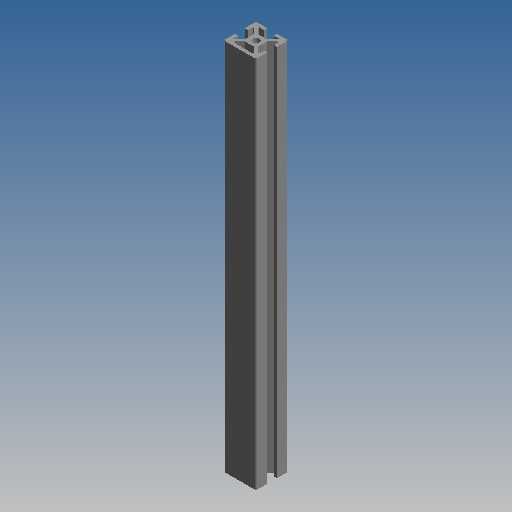
# Autodesk Inventor part: NFSF5-2020-231
Saved by Autodesk Inventor 2020 (Build 240168000, 168)
## iProperties
Part Number: NFSF5-2020-231
Material: 一般
Catalog Web Link: www.cadenas.de
Description: NFS5-2020, NFSB5-2020, HFS5-2020, HFSB5-2020, CAF5-2020, HFSY5-2020, NFSF5-2020, HFSF5-2020, HFSFB5-2020, NFST5-2020, HFST5-2020, HFSTB5-2020, HFSH5-2020, HFSC5-2020-HFS5 Series Aluminum Extrusions 20 Square -1 Slot-
Vendor: MISUMI
Document SubType Name: Modeling
Designer: partserver
Manufacturer: MISUMI
Mass: 44.7598 g
Surface Area: 422.721 cm^2
Volume: 44.7598 cm^3
Density: 1 g/cm^3
Appearance: PSOLRGB-175-175-175
Category: PARTsolutions
Company: MISUMI
PSOL_IDENT_0: {$CADENAS_DATA\23d-libs\misumi\metric\38_al_extrusions_blackets\5\hfs5_2020.prj},678 {VTYP=3D},{NB=N
PSOL_IDENT_1: FSF5-2020-231},{LINA=NFSF5-2020-231},{NN=NFS5-2020, NFSB5-2020, HFS5-2020, HFSB5-2020, CAF5-2020, HF
PSOL_IDENT_2: SY5-2020, NFSF5-2020, HFSF5-2020, HFSFB5-2020, NFST5-2020, HFST5-2020, HFSTB5-2020, HFSH5-2020, HFSC
PSOL_IDENT_3: 5-2020},{DATE=09.09.2019 15:28:27},{GEOMDATE=18.06.2019 07:59:14},{VERSION=},{LINEID=40},{WBVAR=L,AL
PSOL_IDENT_4: T1,ALT2,ALT4,ALT5,CP5,DL5,DR5,ALT6,ALT9,ALT10,ALT11,HP6,NHL6,DL6,NHR6,DR6,ALT7,ALT8,NH9,AH,BH,CH,DH,
PSOL_IDENT_5: EH,NH10,AV,BV,CV,DV,EV,NH11,AP,BP,CP,DP,EP,ALT12,ALT13,Z,NH12,XA,XB,XC,XD,XE,NH13,YA,YB,YC,YD,YE,ALT
PSOL_IDENT_6: 16,HP16,DL16,DR16,ALT17,HQ17,JLP,ALT20},{WBNUMERIC=L,NH9,AH,BH,CH,DH,EH,NH10,AV,BV,CV,DV,EV,NH11,AP,
PSOL_IDENT_7: BP,CP,DP,EP,NH12,XA,XB,XC,XD,XE,NH13,YA,YB,YC,YD,YE,HQ17,JLP}  {NB=NFSF5-2020-231},{LINA=NFSF5-2020-
PSOL_IDENT_8: 231},{KT=DUMMY},{PN=NFSF5-2020-231},{TPS=NFSF5-2020},{MAT=6063-T5 Aluminum Alloy},{ST=Clear Anodize}
PSOL_IDENT_9: ,{FRMW=20},{FRMH=20},{FRD=4.2},{L=231},{MASS=0.53},{SA=195},{LX=0.834x10^4},{LY=0.746x10^4},{ALT1=},
PSOL_IDENT_10: {M1=0},{DPL1=0},{DPR1=0},{ALT1PN=},{ALT2=},{ALT2ALG= '','w/o End Tapping (Heli-Coil Insert)','LHP','
PSOL_IDENT_11: with LHP (Tapping on the Left (Heli-Coil Insert))','RHP','with RHP (Tapping on the Right (Heli-Coil
PSOL_IDENT_12: Insert))','HPW','with HPW (Tapping on Both Ends (Heli-Coil Insert))' },{M2=0},{DP2=0},{ALT2PN=},{ALT
PSOL_IDENT_13: 4=},{ALT4ALG= '', 'w/o SC (High Precision Cut)', 'SC', 'with SC (High Precision Cut)' },{ALT4PN=},{A
PSOL_IDENT_14: LT5=},{ALT5ALG= '','w/o 45 Degree Cut','1','with 45 Degree Cut' },{CP5=},{CP5ALG= '','N/A' },{DL5=},
PSOL_IDENT_15: {DL5ALG= '','N/A' },{DR5=},{DR5ALG= '','N/A' },{FRMLALT5=0},{FRMRALT5=0},{ALT5PN=},{ALT6=},{ALT6ALG=
PSOL_IDENT_16: '','w/o Fastening Location Wrench Access Hole Alterations','1','with Fastening Location Wrench Acce
PSOL_IDENT_17: ss Hole Alterations' },{ALT9=},{ALT9ALG= '','w/o Location Specified Wrench Access Hole Alteratons (H
PSOL_IDENT_18: orizontal)','1','with Location Specified Wrench Access Hole Alteratons (Horizontal)' },{ALT10=},{ALT
PSOL_IDENT_19: 10ALG= '','w/o Location Specified Wrench Access Hole Alteratons (Vertical)','1','with Location Speci
PSOL_IDENT_20: fied Wrench Access Hole Alteratons (Vertical)' },{ALT11=},{ALT11ALG= '','w/o Location Specified Wren
PSOL_IDENT_21: ch Access Hole Alteratons (Crisscross)','1','with Location Specified Wrench Access Hole Alteratons (
PSOL_IDENT_22: Crisscross)' },{HP6=},{HP6ALG= '','N/A' },{NHL6=},{NHL6ALG= '','N/A' },{DL6=},{DL6ALG= '','N/A' },{N
PSOL_IDENT_23: HR6=},{NHR6ALG= '','N/A' },{DR6=},{DR6ALG= '','N/A' },{HL6=0.000},{HL6D=0},{HR6=0.000},{HR6D=0},{J6=
PSOL_IDENT_24: 0},{J6D=0},{K6=0},{K6D=0},{DD6=0.00},{DD6ALG=0},{ALT7=},{ALT7ALG= '','N/A' },{ALT8=},{ALT8ALG= '','N
PSOL_IDENT_25: /A' },{ALT678PN=},{NH9=0},{NH9MAX=5},{NH9ALG=[0]},{AH=0.0},{AHMIN=7},{AHMAX=226},{AHALG=[0]},{BH=0.0
PSOL_IDENT_26: },{BHMIN=2},{BHMAX=228},{BHALG=[0]},{CH=0.0},{CHMIN=2},{CHMAX=230},{CHALG=[0]},{DH=0.0},{DHMIN=2},{D
PSOL_IDENT_27: HMAX=232},{DHALG=[0]},{EH=0.0},{EHMIN=2},{EHMAX=224},{EHALG=[0]},{NH10=0},{NH10MAX=5},{NH10ALG=[0]},
PSOL_IDENT_28: {AV=0.0},{AVMIN=7},{AVMAX=226},{AVALG=[0]},{BV=0.0},{BVMIN=2},{BVMAX=228},{BVALG=[0]},{CV=0.0},{CVMI
PSOL_IDENT_29: N=2},{CVMAX=230},{CVALG=[0]},{DV=0.0},{DVMIN=2},{DVMAX=232},{DVALG=[0]},{EV=0.0},{EVMIN=2},{EVMAX=22
PSOL_IDENT_30: 4},{EVALG=[0]},{NH11=0},{NH11MAX=5},{NH11ALG=[0]},{AP=0.0},{APMIN=7},{APMAX=226},{APALG=[0]},{BP=0.0
PSOL_IDENT_31: },{BPMIN=2},{BPMAX=228},{BPALG=[0]},{CP=0.0},{CPMIN=2},{CPMAX=230},{CPALG=[0]},{DP=0.0},{DPMIN=2},{D
PSOL_IDENT_32: PMAX=232},{DPALG=[0]},{EP=0.0},{EPMIN=2},{EPMAX=224},{EPALG=[0]},{ALT9PN=},{ALT10PN=},{ALT11PN=},{AL
PSOL_IDENT_33: T91011PN=},{ALT12=},{ALT12ALG= '','w/o Counterbore Hole in Specified Position (Vertical)','1','with
PSOL_IDENT_34: Counterbore Hole in Specified Position (Vertical)' },{ALT13=},{ALT13ALG= '','w/o Counterbore Hole in
PSOL_IDENT_35: Specified Position (Horizontal)','1','with Counterbore Hole in Specified Position (Horizontal)' },{
PSOL_IDENT_36: Z=},{ZALG= '','N/A' },{DD12=0.0},{DD112=0.0},{NH12=0},{NH12MAX=5},{NH12ALG=[0]},{XA=0.0},{XAMIN=7},{
PSOL_IDENT_37: XAMAX=226},{XAALG=[0]},{XB=0.0},{XBMIN=2},{XBMAX=228},{XBALG=[0]},{XC=0.0},{XCMIN=2},{XCMAX=230},{XC
PSOL_IDENT_38: ALG=[0]},{XD=0.0},{XDMIN=2},{XDMAX=232},{XDALG=[0]},{XE=0.0},{XEMIN=2},{XEMAX=224},{XEALG=[0]},{NH13=
PSOL_IDENT_39: 0},{NH13MAX=5},{NH13ALG=[0]},{YA=0.0},{YAMIN=7},{YAMAX=226},{YAALG=[0]},{YB=0.0},{YBMIN=2},{YBMAX=22
PSOL_IDENT_40: 8},{YBALG=[0]},{YC=0.0},{YCMIN=2},{YCMAX=230},{YCALG=[0]},{YD=0.0},{YDMIN=2},{YDMAX=232},{YDALG=[0]}
PSOL_IDENT_41: ,{YE=0.0},{YEMIN=2},{YEMAX=224},{YEALG=[0]},{ALT12PN=},{ALT13PN=},{ALT1213PN=},{ALT16=},{ALT16ALG= ''
PSOL_IDENT_42: ,'w/o M Type Hole Alteration','1','with M Type Hole Alteration' },{HP16=},{HP16ALG= '','N/A' },{DL16=
PSOL_IDENT_43: },{DL16ALG= '','N/A' },{DR16=},{DR16ALG= '','N/A' },{H116=0},{D16=0.0},{ALT16PN=},{ALT17=},{ALT17ALG=
PSOL_IDENT_44: '','w/o L Type Hole Alteration (Top)','1','with L Type Hole Alteration (Top)' },{HQ17=0},{HQ17ALG=0
PSOL_IDENT_45: },{JLP=0},{JLPMIN=4.9},{JLPMAX=0},{JLPALG=[0]},{L17=0},{D17=0.0},{ALT17PN=},{ALT20=},{ALT20PN=},{ERR
PSOL_IDENT_46: ORALT01=OK},{ERRORALT02=OK},{ERRORALT05=OK},{ERRORALT06091=OK},{ERRORALT06092=OK},{ERRORALT06093=OK}
PSOL_IDENT_47: ,{ERRORALT06094=OK},{ERRORALT06101=OK},{ERRORALT06102=OK},{ERRORALT06103=OK},{ERRORALT06104=OK},{ERR
PSOL_IDENT_48: ORALT06111=OK},{ERRORALT06112=OK},{ERRORALT06113=OK},{ERRORALT06114=OK},{ERRORALT06121=OK},{ERRORALT
PSOL_IDENT_49: 06122=OK},{ERRORALT06123=OK},{ERRORALT06124=OK},{ERRORALT06131=OK},{ERRORALT06132=OK},{ERRORALT06133=
PSOL_IDENT_50: OK},{ERRORALT06134=OK},{ERRORALT0616=OK},{ERRORALT06171=OK},{ERRORALT06172=OK},{ERRORALT06173=OK},{E
PSOL_IDENT_51: RRORALT0911=OK},{ERRORALT0913=OK},{ERRORALT0916=OK},{ERRORALT0917=OK},{ERRORALT1011=OK},{ERRORALT101
PSOL_IDENT_52: 2=OK},{ERRORALT1016=OK},{ERRORALT1017=OK},{ERRORALT1112=OK},{ERRORALT1113=OK},{ERRORALT1116=OK},{ERR
PSOL_IDENT_53: ORALT1117=OK},{ERRORALT1216=OK},{ERRORALT1217=OK},{ERRORALT1316=OK},{ERRORALT1317=OK},{ERRORALT1617=
PSOL_IDENT_54: OK},{ERRORPN=},{TFW=0}
NB: NFSF5-2020-231
NN: NFS5-2020, NFSB5-2020, HFS5-2020, HFSB5-2020, CAF5-2020, HFSY5-2020, NFSF5-2020, HFSF5-2020, HFSFB5-2020, NFST5-2020, HFST5-2020, HFSTB5-2020, HFSH5-2020, HFSC5-2020
NT: HFS5 Series Aluminum Extrusions 20 Square -1 Slot-
NBSYN: $PN.
LINA: NFSF5-2020-231
CATALOG: Misumi
PN: NFSF5-2020-231
TPS: NFSF5-2020
MAT: 6063-T5 Aluminum Alloy
ST: Clear Anodize
L: 231
MASS: 0.53
SA: 195
LX: 0.834x10^4
LY: 0.746x10^4
ALT1: w/o End Tapping
M1: 0
DPL1: 0
DPR1: 0
ALT2: w/o End Tapping (Heli-Coil Insert)
M2: 0
DP2: 0
ALT4: w/o SC (High Precision Cut)
ALT5: w/o 45 Degree Cut
CP5: N/A
DL5: N/A
DR5: N/A
ALT6: w/o Fastening Location Wrench Access Hole Alterations
ALT9: w/o Location Specified Wrench Access Hole Alteratons (Horizontal)
ALT10: w/o Location Specified Wrench Access Hole Alteratons (Vertical)
ALT11: w/o Location Specified Wrench Access Hole Alteratons (Crisscross)
HP6: N/A
NHL6: N/A
DL6: N/A
NHR6: N/A
DR6: N/A
HL6D: 0
HR6D: 0
J6D: 0
K6D: 0
DD6: 0
ALT7: N/A
ALT8: N/A
NH9: 0
AH: 0
BH: 0
CH: 0
DH: 0
EH: 0
NH10: 0
AV: 0
BV: 0
CV: 0
DV: 0
EV: 0
NH11: 0
AP: 0
BP: 0
CP: 0
DP: 0
EP: 0
ALT12: w/o Counterbore Hole in Specified Position (Vertical)
ALT13: w/o Counterbore Hole in Specified Position (Horizontal)
Z: N/A
DD12: 0
DD112: 0
NH12: 0
XA: 0
XB: 0
XC: 0
XD: 0
XE: 0
NH13: 0
YA: 0
YB: 0
YC: 0
YD: 0
YE: 0
ALT16: w/o M Type Hole Alteration
HP16: N/A
DL16: N/A
DR16: N/A
H116: 0
D16: 0
ALT17: w/o L Type Hole Alteration (Top)
HQ17: 0
JLP: 0
D17: 0
ALT20: w/o CW (End Face C Chamfering)
SUPPLIER: MISUMI
ARTICLENO: NFSF5-2020-231
BOMINFO: NFSF5-2020-231
CREATOR: CADENAS GmbH
Title: NFSF5-2020-231
Author: Cadenas PARTsolutions
Comments: HFS5 Series Aluminum Extrusions 20 Square -1 Slot-
Autodesk Inventor part; units mm, degrees
sketch "Sketch_76" plane through (0, 0, 0) normal (0, 0, 1) x (1, 0, 0)
  line L0 (-10, -3) -> (-10, -9)
  arc A0 (-10, -9) -> (-9, -10) centre (-9, -9) ccw
  line L1 (-9, -10) -> (9, -10)
  arc A1 (9, -10) -> (10, -9) centre (9, -9) ccw
  line L2 (10, -9) -> (10, -3)
  line L3 (10, -3) -> (8, -3)
  line L4 (8, -3) -> (8, -6)
  line L5 (8, -6) -> (7.0607, -6)
  line L6 (7.0607, -6) -> (4, -2.9393)
  line L7 (4, -2.9393) -> (4, -0.6536)
  arc A2 (4, -0.6536) -> (3.933, -0.4036) centre (3.5, -0.6536) ccw
  line L8 (3.933, -0.4036) -> (3.7, 0)
  line L9 (3.7, 0) -> (3.933, 0.4036)
  arc A3 (3.933, 0.4036) -> (3.933, 0.9036) centre (3.5, 0.6536) ccw
  line L10 (3.933, 0.9036) -> (3.751, 1.2189)
  line L11 (3.751, 1.2189) -> (4, 2.5)
  line L12 (4, 2.5) -> (4, 2.9393)
  line L13 (4, 2.9393) -> (7.0607, 6)
  line L14 (7.0607, 6) -> (8, 6)
  line L15 (8, 6) -> (8, 3)
  line L16 (8, 3) -> (10, 3)
  line L17 (10, 3) -> (10, 9)
  arc A4 (10, 9) -> (9, 10) centre (9, 9) ccw
  line L18 (9, 10) -> (3, 10)
  line L19 (3, 10) -> (3, 8)
  line L20 (3, 8) -> (6, 8)
  line L21 (6, 8) -> (6, 7.0607)
  line L22 (6, 7.0607) -> (2.9393, 4)
  line L23 (2.9393, 4) -> (0.6536, 4)
  arc A5 (0.6536, 4) -> (0.4036, 3.933) centre (0.6536, 3.5) ccw
  line L24 (0.4036, 3.933) -> (0, 3.7)
  line L25 (0, 3.7) -> (-0.4036, 3.933)
  arc A6 (-0.4036, 3.933) -> (-0.9036, 3.933) centre (-0.6536, 3.5) ccw
  line L26 (-0.9036, 3.933) -> (-1.2189, 3.751)
  line L27 (-1.2189, 3.751) -> (-2.5, 4)
  line L28 (-2.5, 4) -> (-2.9393, 4)
  line L29 (-2.9393, 4) -> (-6, 7.0607)
  line L30 (-6, 7.0607) -> (-6, 8)
  line L31 (-6, 8) -> (-3, 8)
  line L32 (-3, 8) -> (-3, 10)
  line L33 (-3, 10) -> (-9, 10)
  arc A7 (-9, 10) -> (-10, 9) centre (-9, 9) ccw
  line L34 (-10, 9) -> (-10, 3)
  line L35 (-10, 3) -> (-8, 3)
  line L36 (-8, 3) -> (-8, 6)
  line L37 (-8, 6) -> (-7.0607, 6)
  line L38 (-7.0607, 6) -> (-4, 2.9393)
  line L39 (-4, 2.9393) -> (-4, 0.6536)
  arc A8 (-4, 0.6536) -> (-3.933, 0.4036) centre (-3.5, 0.6536) ccw
  line L40 (-3.933, 0.4036) -> (-3.7, 0)
  line L41 (-3.7, 0) -> (-3.933, -0.4036)
  arc A9 (-3.933, -0.4036) -> (-3.933, -0.9036) centre (-3.5, -0.6536) ccw
  line L42 (-3.933, -0.9036) -> (-3.751, -1.2189)
  line L43 (-3.751, -1.2189) -> (-4, -2.5)
  line L44 (-4, -2.5) -> (-4, -2.9393)
  line L45 (-4, -2.9393) -> (-7.0607, -6)
  line L46 (-7.0607, -6) -> (-8, -6)
  line L47 (-8, -6) -> (-8, -3)
  line L48 (-8, -3) -> (-10, -3)
  line L49 (-6, -7.2678) -> (-6, -7.5)
  arc A10 (-6, -7.5) -> (-5.5, -8) centre (-5.5, -7.5) ccw
  line L50 (-5.5, -8) -> (5.5, -8)
  arc A11 (5.5, -8) -> (6, -7.5) centre (5.5, -7.5) ccw
  line L51 (6, -7.5) -> (6, -7.2678)
  arc A12 (6, -7.2678) -> (5.8536, -6.9142) centre (5.5, -7.2678) ccw
  line L52 (5.8536, -6.9142) -> (3.0858, -4.1464)
  arc A13 (3.0858, -4.1464) -> (2.7322, -4) centre (2.7322, -4.5) ccw
  line L53 (2.7322, -4) -> (-2.7322, -4)
  arc A14 (-2.7322, -4) -> (-3.0858, -4.1464) centre (-2.7322, -4.5) ccw
  line L54 (-3.0858, -4.1464) -> (-5.8536, -6.9142)
  arc A15 (-5.8536, -6.9142) -> (-6, -7.2678) centre (-5.5, -7.2678) ccw
  constraints: 110 end point, 32 point on circle, 16 centre point
extrude "Extrusion1" add sketch "Sketch_76" against normal blind 231
sketch "Sketch2" plane through (0, 0, -231) normal (0, 0, -1) x (-1, 0, 0)
  point P0 (0, 0)
hole "Hole1" at (0, 0, -231) direction (0, 0, 1) diameter 4.2 depth 231
ref_plane "C1_XY" through (0, 0, 0) normal (0, 0, 1) x (1, 0, 0)
ref_plane "C1_YZ" through (0, 0, 0) normal (1, 0, 0) x (0, 1, 0)
ref_plane "C1_ZX" through (0, 0, 0) normal (0, 1, 0) x (0, 0, 1)
body "Solid1"
